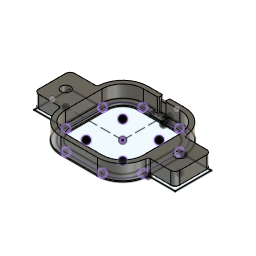
50kg_Loadcell_Bracket (Autodesk Fusion 360 design; units mm, degrees)
Autodesk Fusion 360 part; units mm, degrees
sketch "Sketch1" plane through (0, 0, 0) normal (0, 0, 1) x (1, 0, 0) in component "inside"
  line L0 (8.1, -17.1) -> (-8.1, -17.1)
  line L1 (-17.1, -8.1) -> (-17.1, 8.1)
  line L2 (-8.1, 17.1) -> (8.1, 17.1)
  line L3 (17.1, 8.1) -> (17.1, -8.1)
  line L4 (17.1, -17.1) -> (-17.1, 17.1) construction
  line L5 (-17.1, -17.1) -> (17.1, 17.1) construction
  arc A0 (-8.1, 17.1) -> (-17.1, 8.1) centre (-8.1, 8.1) ccw
  arc A1 (17.1, 8.1) -> (8.1, 17.1) centre (8.1, 8.1) ccw
  arc A2 (8.1, -17.1) -> (17.1, -8.1) centre (8.1, -8.1) ccw
  arc A3 (-17.1, -8.1) -> (-8.1, -17.1) centre (-8.1, -8.1) ccw
  arc A4 (-8.1, 14.1) -> (-14.1, 8.1) centre (-8.1, 8.1) ccw
  line L6 (-14.1, -8.1) -> (-14.1, 8.1)
  arc A5 (-14.1, -8.1) -> (-8.1, -14.1) centre (-8.1, -8.1) ccw
  line L7 (8.1, -14.1) -> (-8.1, -14.1)
  arc A6 (8.1, -14.1) -> (14.1, -8.1) centre (8.1, -8.1) ccw
  line L8 (14.1, 8.1) -> (14.1, -8.1)
  arc A7 (14.1, 8.1) -> (8.1, 14.1) centre (8.1, 8.1) ccw
  line L9 (-8.1, 14.1) -> (8.1, 14.1)
  line L10 (-17.1, 0) -> (17.1, 0) construction
  line L11 (0, 17.1) -> (0, -17.5036) construction
  dimension "d1" = 34.2
  dimension "d2" = 34.2
  dimension "d3" = 9
  dimension "d4" = 3
  constraint horizontal L0
  constraint perpendicular L0 L1
  constraint parallel L0 L2
  constraint parallel L1 L3
  constraint coincident L4 origin
  constraint coincident L5 origin
  constraint coincident L4.end L1
  constraint coincident L4.end L2
  constraint tangent L1 A0
  constraint tangent L2 A0
  constraint coincident L5.end L2
  constraint coincident L5.end L3
  constraint tangent L2 A1
  constraint tangent L3 A1
  constraint equal A0 A1
  constraint coincident L4.start L3
  constraint coincident L4.start L0
  constraint tangent L3 A2
  constraint tangent L0 A2
  constraint equal A0 A2
  constraint coincident L5.start L0
  constraint coincident L5.start L1
  constraint tangent L0 A3
  constraint tangent L1 A3
  constraint equal A0 A3
  constraint midpoint L1 L10.start
  constraint midpoint L3 L10.end
  constraint midpoint L2 L11.start
  constraint perpendicular L0 L11
  measures "d1" distance of L4.end L5.end
  measures "d2" distance of L5.start L4.end
  measures "d3" radius of A0
extrude "Extrude1" add sketch "Sketch1" along normal blind 3 makes body 1 in component "inside"
sketch "Sketch1 (2)" plane through (0, 0, 0) normal (0, 0, 1) x (1, 0, 0) in component "outside"
  arc A0 (-8.1, 17.1) -> (-17.1, 8.1) centre (-8.1, 8.1) ccw
  line L0 (-8.1, 17.1) -> (8.1, 17.1)
  arc A1 (17.1, 8.1) -> (8.1, 17.1) centre (8.1, 8.1) ccw
  line L1 (17.1, 8.1) -> (17.1, -8.1)
  arc A2 (8.1, -17.1) -> (17.1, -8.1) centre (8.1, -8.1) ccw
  line L2 (8.1, -17.1) -> (-8.1, -17.1)
  arc A3 (-17.1, -8.1) -> (-8.1, -17.1) centre (-8.1, -8.1) ccw
  line L3 (-17.1, -8.1) -> (-17.1, 8.1)
  arc A4 (-8.1, 17.3) -> (-17.3, 8.1) centre (-8.1, 8.1) ccw
  line L4 (-17.3, -8.1) -> (-17.3, 8.1)
  arc A5 (-17.3, -8.1) -> (-8.1, -17.3) centre (-8.1, -8.1) ccw
  line L5 (8.1, -17.3) -> (-8.1, -17.3)
  arc A6 (8.1, -17.3) -> (17.3, -8.1) centre (8.1, -8.1) ccw
  line L6 (17.3, 8.1) -> (17.3, -8.1)
  arc A7 (17.3, 8.1) -> (8.1, 17.3) centre (8.1, 8.1) ccw
  line L7 (-8.1, 17.3) -> (8.1, 17.3)
  arc A8 (-8.1, 19.3) -> (-19.3, 8.1) centre (-8.1, 8.1) ccw
  line L8 (-19.3, -8.1) -> (-19.3, 8.1)
  arc A9 (-19.3, -8.1) -> (-8.1, -19.3) centre (-8.1, -8.1) ccw
  line L9 (8.1, -19.3) -> (-8.1, -19.3)
  arc A10 (8.1, -19.3) -> (19.3, -8.1) centre (8.1, -8.1) ccw
  line L10 (19.3, 8.1) -> (19.3, -8.1)
  arc A11 (19.3, 8.1) -> (8.1, 19.3) centre (8.1, 8.1) ccw
  line L11 (-8.1, 19.3) -> (8.1, 19.3)
  line L12 (-15.1, -8.1) -> (-15.1, 8.1)
  arc A12 (-8.1, 15.1) -> (-15.1, 8.1) centre (-8.1, 8.1) ccw
  line L13 (-8.1, 15.1) -> (8.1, 15.1)
  arc A13 (15.1, 8.1) -> (8.1, 15.1) centre (8.1, 8.1) ccw
  line L14 (15.1, 8.1) -> (15.1, -8.1)
  arc A14 (8.1, -15.1) -> (15.1, -8.1) centre (8.1, -8.1) ccw
  line L15 (8.1, -15.1) -> (-8.1, -15.1)
  arc A15 (-15.1, -8.1) -> (-8.1, -15.1) centre (-8.1, -8.1) ccw
  line L16 (0, 0) -> (-31.3, 0) construction
  line L17 (-19.3, 8) -> (-31.3, 8)
  line L18 (-31.3, 8) -> (-31.3, -8)
  line L19 (-31.3, -8) -> (-19.3, -8)
  line L20 (0, 0) -> (0, 24) construction
  line L21 (19.3, 8) -> (31.3, 8)
  line L22 (31.3, -8) -> (19.3, -8)
  line L23 (31.3, 8) -> (31.3, -8)
  line L24 (-3, 15.1) -> (-3, 17.3)
  line L25 (-1.5, 17.3) -> (-1.5, 19.3)
  line L26 (1.5, 17.3) -> (1.5, 19.3)
  line L27 (3, 15.1) -> (3, 17.3)
  line L28 (-1.5, 18.5) -> (1.5, 18.5)
  point P0 (-25.3, 0)
  point P1 (25.3, 0)
  dimension "d10" = 0.2
  dimension "d11" = -2.2
  dimension "d14" = 2
  dimension "d15" = 12
  dimension "d16" = 8
  dimension "d17" = 16
  dimension "d18" = 6
  dimension "d20" = 3
  dimension "d21" = 1.5
  dimension "d26" = 0.8
  constraint coincident L16.start L20.start
  constraint horizontal L16
  constraint coincident L8 L17.start
  constraint perpendicular L8 L17
  constraint perpendicular L17 L18
  constraint coincident L8 L19.end
  constraint perpendicular L8 L19
  constraint coincident L16 P0
  constraint perpendicular L16 L20
  constraint symmetric L17.start L20 L21.start
  constraint symmetric L17.end L20 L21.end
  constraint symmetric L18.end L20 L22.start
  constraint symmetric L19.end L20 L22.end
  constraint symmetric P0 L20 P1
  constraint coincident L13 L24.start
  constraint coincident L7 L24.end
  constraint perpendicular L7 L24
  constraint coincident L7 L25.start
  constraint coincident L11 L25.end
  constraint perpendicular L11 L25
  constraint symmetric L20 L24.start L27.start
  constraint symmetric L20 L24.end L27.end
  constraint symmetric L20 L25.start L26.start
  constraint symmetric L20 L25.end L26.end
  constraint coincident L25 L28.start
  constraint coincident L26 L28.end
  constraint perpendicular L26 L28
  measures "d15" distance of L17.start L17.end
  measures "d16" distance of L16 L17
  measures "d17" distance of L17.end L18.end
  measures "d18" distance of L18 P0
  measures "d20" distance of L20 L24
  measures "d21" distance of L20 L25
  measures "d26" distance of L11 L28
extrude "Extrude1'" add sketch "Sketch1 (2)" along normal blind 7 separate body contours A4 L4 A5 L5 A6 L6 A7 L7 A8 L8 A9 L9 A10 L10 A11 L11 L25 L26 | L7 L25 L26 L28 | L11 L25 L26 L28 makes body 2 in component "outside"
extrude "Extrude2" add sketch "Sketch1 (2)" along normal blind 1.5 contours A0 L0 A1 L1 A2 L2 A3 L3 L12 A12 L13 A13 L14 A14 L15 A15 L24 L27 | A0 L0 A1 L1 A2 L2 A3 L3 A4 L4 A5 L5 A6 L6 A7 L7 L24 L27 bodies 2 in component "outside"
extrude "Extrude3" add sketch "Sketch1 (2)" along normal blind 0.8 contours L0 L7 L24 L27 | L0 L13 L24 L27 bodies 2 in component "outside"
extrude "Extrude4" cut sketch "Sketch1 (2)" along normal up to surface (6.2 mm away) from surface at 0.8 contours L7 L25 L26 L28 bodies 2 in component "outside"
extrude "Extrude5" cut sketch "Sketch1 (2)" against normal blind 1.5 from surface at 7 contours L11 L25 L26 L28 bodies 2 in component "outside"
extrude "Extrude6" add sketch "Sketch1 (2)" against normal blind 6 from surface at 7 contours L8 L17 L18 L19 | L10 L21 L22 L23 bodies 2 in component "outside"
sketch "Sketch2" plane through (0, 0, 1) normal (0, 0, -1) x (1, 0, 0) in component "outside"
  line L0 (19.3, -8) -> (31.3, -8)
  line L1 (31.3, -8) -> (31.3, 8)
  line L2 (31.3, 8) -> (19.3, 8)
  line L3 (19.3, 8) -> (19.3, -8)
  point P0 (25.3, 0)
  point P1 (-25.3, 0)
  point P2 (25.3, 0)
  point P3 (-25.3, 0)
  constraint coincident P2 P0
  constraint coincident P3 P1
hole "Hole2" at (25.3, 0, 1) at (-25.3, 0, 1) direction (0, 0, 1) diameter 4.17 end up to surface (6 mm away) countersink diameter 8.43 countersink angle 84 bodies 2 in component "outside"
fillet "Fillet1" radius 0.4 1 faces at (-2.7, -16.5, 0) on bodies 2 in component "outside"
fillet "Fillet2" radius 2 4 edges at (-31.3, 8, 4) (-31.3, -8, 4) (31.3, 8, 4) (31.3, -8, 4) on bodies 2 in component "outside"
fillet "Fillet3" radius 1 4 edges at (19.3, -8, 4) (19.3, 8, 4) (-19.3, -8, 4) (-19.3, 8, 4) on bodies 2 in component "outside"
fillet "Fillet4" radius 0.4 20 edges at (-19.5862, -8.2673, 1) (-24.7834, -8, 1) (-30.7142, -7.4142, 1) (-31.3, 0, 1) (-30.7142, 7.4142, 1) (-24.7834, 8, 1) (-19.5862, 8.2673, 1) (19.5862, 8.2673, 1) (24.7834, 8, 1) (30.7142, 7.4142, 1) (31.3, 0, 1) (30.7142, -7.4142, 1) (24.7834, -8, 1) (19.5862, -8.2673, 1) (-1.5, 19.3, 6.25) (0, 19.3, 5.5) (1.5, 19.3, 6.25) (1.5, 17.3, 3.9) (-1.5, 17.3, 3.9) (0, 18.5, 5.5) on bodies 2 in component "outside"
move_body "Move1" bodies 1 to x (1, 0, 0) y (0, 1, 0) z (0, 0, 1) at (50, 0, 0) in component "inside"
component "inside" placed x (1, 0, 0) y (0, 1, 0) z (0, 0, 1) at (0, 0, 0)
component "outside" placed x (1, 0, 0) y (0, 1, 0) z (0, 0, 1) at (0, 0, 0)
equation "d11 = -0.2 mm - 2 mm"
named bodies: "inside", "outside"
